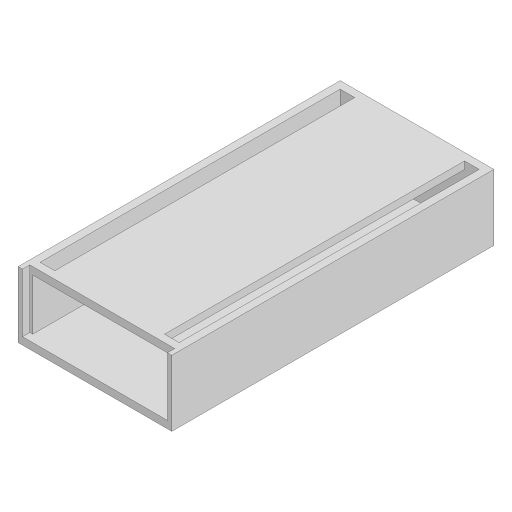
# Autodesk Inventor part: Team29_PiBox
Saved by Autodesk Inventor 2023 (Build 270158000, 158)
## iProperties
Created: 2023-02-27
Part Number: Team29_PiBox
Material: Generic
Document SubType Name: Modeling
Designer: Fariha
Density: 1 g/cm^3
Appearance: Default
Author: Fariha
Autodesk Inventor part; units mm, degrees
ref_plane "YZ Plane" through (0, 0, 0) normal (1, 0, 0) x (0, 1, 0)
ref_plane "XZ Plane" through (0, 0, 0) normal (0, 1, 0) x (-1, 0, 0)
ref_plane "XY Plane" through (0, 0, 0) normal (0, 0, 1) x (1, 0, 0)
sketch "Sketch2" plane through (0, 0, 0) normal (0, 0, 1) x (1, 0, 0)
  line L0 (-47.5, 20) -> (47.5, 20)
  line L1 (47.5, 20) -> (47.5, -25)
  line L2 (47.5, -25) -> (-47.5, -25)
  line L3 (-47.5, -25) -> (-47.5, 20)
  line L4 (-52.5, 20) -> (52.5, 20)
  line L5 (52.5, 20) -> (52.5, -25)
  line L6 (52.5, -25) -> (-52.5, -25)
  line L7 (-52.5, -25) -> (-52.5, 20)
  line L8 (-47.5, 15) -> (47.5, 15)
  line L9 (47.5, 15) -> (47.5, -20)
  line L10 (47.5, -20) -> (-47.5, -20)
  line L11 (-47.5, -20) -> (-47.5, 15)
  point P0 (0, 0)
  dimension "d4" = 95
  dimension "d5" = 45
  dimension "d6" = 47.5
  dimension "d7" = 20
  dimension "d8" = 5
  dimension "d9" = 5
  dimension "d10" = 5
  dimension "d11" = 5
  dimension "d12" = 45
  dimension "d13" = 5
  constraints: 24 end point, 6 parallel, 3 horizontal, 3 perpendicular, 2 point on line
  measures "d4" distance of L1.end L2.end
  measures "d5" distance of L0.end L1.end
  measures "d6" distance from line of L3 point (0, 0)
  measures "d7" distance from line of L0 point (0, 0)
  measures "d8" distance between parallel lines of L7 L3
  measures "d9" distance between parallel lines of L1 L5
  measures "d10" distance between parallel lines of L0 L8
  measures "d11" distance between parallel lines of L2 L10
  measures "d12" distance between parallel lines of L4 L6
  measures "d13" distance between parallel lines of L8 L4
extrude "Extrusion1" add sketch "Sketch2" against normal blind 210 contours L0 L1 L8 L3 | L3 L6 L7 L4 | L4 L5 L6 L1 | L10 L1 L2 L3
sketch "Sketch3" plane through (0, 0, -210) normal (0, 0, -1) x (-1, 0, 0)
  point P0 (0, 0)
sketch "Sketch4" plane through (0, 0, -210) normal (0, 0, -1) x (-1, 0, 0)
  line L0 (-52.5, -25) -> (-52.5, 20) projected
  line L1 (52.5, -25) -> (-52.5, -25) projected
  line L2 (-52.5, 20) -> (52.5, 20)
  line L3 (52.5, 20) -> (52.5, -25)
  line L4 (52.5, -25) -> (-52.5, -25)
  line L5 (-52.5, -25) -> (-52.5, 20)
  point P0 (0, 0)
  constraints: 8 end point, 2 parallel, 1 horizontal, 1 perpendicular
extrude "Extrusion2" add sketch "Sketch4" along normal blind 5
sketch "Sketch8" plane through (-52.5, 20, -215) normal (0, 1, 0) x (1, 0, 0)
  line L0 (5, -215) -> (5, -5) projected
  line L1 (5, -5) -> (15, -5)
  line L2 (15, -5) -> (15, -210)
  line L3 (15, -210) -> (5, -210)
  line L4 (5, -210) -> (5, -5)
  line L5 (100, -215) -> (100, -5) projected
  line L6 (100, -5) -> (90, -5)
  line L7 (90, -5) -> (90, -210)
  line L8 (90, -210) -> (100, -210)
  line L9 (100, -210) -> (100, -5)
  point P0 (52.5, -215)
  point P1 (100, -210)
  dimension "d33" = 10
  dimension "d34" = 205
  dimension "d35" = 10
  constraints: 16 end point, 4 parallel, 2 horizontal, 2 perpendicular, 1 point on line
  measures "d33" distance of L2.end L3.end
  measures "d34" distance of L1.end L2.end
  measures "d35" distance of L8.end L7.end
extrude "Extrusion6" cut sketch "Sketch8" against normal blind 5
sketch "Sketch11" plane through (-52.5, -25, 0) normal (0, -1, 0) x (1, 0, 0)
  line L0 (0, 0) -> (0, -215) projected
  line L1 (0, 0) -> (105, 0)
  line L2 (105, 0) -> (105, 5)
  line L3 (105, 5) -> (0, 5)
  line L4 (0, 5) -> (0, 0)
  line L5 (0, 0) -> (105, 0) projected
  line L6 (0, 0) -> (3, 0)
  line L7 (3, 0) -> (3, 5)
  line L8 (3, 5) -> (0, 5)
  line L9 (0, 5) -> (0, 0)
  line L10 (105, 0) -> (102, 0)
  line L11 (102, 0) -> (102, 5)
  line L12 (102, 5) -> (105, 5)
  line L13 (105, 5) -> (105, 0)
  point P0 (52.5, 0)
  point P1 (3, 0)
  dimension "d48" = 5
  dimension "d49" = 3
  dimension "d50" = 3
  constraints: 24 end point, 6 parallel, 3 horizontal, 3 perpendicular, 2 point on line
  measures "d48" distance of L2.end L1.end
  measures "d49" distance of L8.end L7.end
  measures "d50" distance of L11.end L12.end
extrude "Extrusion9" add sketch "Sketch11" against normal blind 5 contours L7 L3 L11 L1
extrude "Extrusion10" add sketch "Sketch11" against normal blind 45 contours L4 L3 L7 L1 | L11 L3 L2 L1
body "Solid1"
